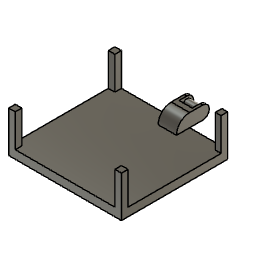
base-plate v2 (Autodesk Fusion 360 design; units mm, degrees)
Autodesk Fusion 360 part; units mm, degrees
sketch "Sketch1" plane through (0, 0, 0) normal (0, 0, 1) x (1, 0, 0)
  line L0 (0, 0) -> (76, 0)
  line L1 (76, 0) -> (76, 76)
  line L2 (76, 76) -> (0, 76)
  line L3 (0, 76) -> (0, 0)
  dimension "d1" = 76
  dimension "d2" = 76
  constraint horizontal L0
  constraint vertical L1
  constraint horizontal L2
  constraint vertical L3
  constraint coincident L0.start L3.end
  measures "d1" distance of L0.start L0.end
  measures "d2" distance of L0.start L2.end
extrude "Extrude1" add sketch "Sketch1" along normal blind 6.35
sketch "Sketch2" plane through (0, 0, 6.35) normal (0, 0, 1) x (-1, 0, 0)
  line L0 (0, -76) -> (0, 0)
  line L1 (0, 0) -> (-76, 0)
  line L2 (-76, 0) -> (-76, -76)
  line L3 (-76, -76) -> (0, -76)
  line L4 (-52, -66) -> (-38, -66)
  line L5 (-38, -66) -> (-38, -91)
  line L6 (-38, -91) -> (-52, -91)
  line L7 (-52, -91) -> (-52, -66)
  dimension "d5" = 14
  dimension "d6" = 25
  dimension "d7" = 24
  dimension "d8" = 10
  constraint horizontal L4
  constraint vertical L5
  constraint horizontal L6
  constraint vertical L7
  measures "d5" distance of L4.start L4.end
  measures "d6" distance of L4.start L6.end
  measures "d7" distance of L2 L7
  measures "d8" distance of L3 L4
extrude "Extrude2" add sketch "Sketch2" along normal blind 10 contours L3 L5 L6 L7 | L3 L4 L5 L7
fillet "Fillet1" radius 10 1 edges at (45, 66, 16.35)
fillet "Fillet2" radius 5 2 edges at (45, 91, 16.35) (45, 91, 6.35)
sketch "Sketch3" plane through (0, 0, 16.35) normal (0, 0, 1) x (-1, 0, 0)
  line L0 (-52, -86) -> (-38, -86)
  line L1 (-38, -86) -> (-38, -76)
  line L2 (-38, -76) -> (-52, -76)
  line L3 (-52, -76) -> (-52, -86)
  line L4 (-50, -80) -> (-40, -80)
  line L5 (-40, -80) -> (-40, -95)
  line L6 (-40, -95) -> (-50, -95)
  line L7 (-50, -95) -> (-50, -80)
  constraint horizontal L4
  constraint vertical L5
  constraint horizontal L6
  constraint vertical L7
extrude "Extrude3" cut sketch "Sketch3" against normal blind 20 contours L0 L4 L5 L7 | L0 L5 L6 L7
sketch "Sketch4" plane through (40, 0, 0) normal (1, 0, 0) x (0, 1, 0)
  line L0 (80, 6.35) -> (86, 6.35)
  arc A0 (86, 6.35) -> (86, 16.35) centre (86, 11.35) ccw
  line L1 (86, 16.35) -> (80, 16.35)
  line L2 (80, 16.35) -> (80, 6.35)
  circle A1 centre (86, 11.35) radius 3.25
  dimension "d17" = 6.5
  constraint concentric A0 A1
  measures "d17" diameter of A1
extrude "Extrude4" add sketch "Sketch4" along normal blind 10 contours A1
extrude "Extrude5" add 1 faces at (76, 25.3333, 2.1167) along direction (1, 0, 0) blind 5
extrude "Extrude6" add 1 faces at (0, 50.6667, 2.1167) along direction (-1, 0, 0) blind 5
extrude "Extrude7" add 1 faces at (23.6667, 0, 2.1167) along direction (0, -1, 0) blind 5
sketch "Sketch5" plane through (0, 0, 6.35) normal (0, 0, 1) x (-1, 0, 0)
  line L0 (-38, -66) -> (-38, -76)
  line L1 (-38, -76) -> (5, -76)
  line L2 (5, -76) -> (5, 5)
  line L3 (5, 5) -> (-81, 5)
  line L4 (-81, 5) -> (-81, -76)
  line L5 (-81, -76) -> (-52, -76)
  line L6 (-52, -76) -> (-52, -66)
  line L7 (-52, -66) -> (-38, -66)
  line L8 (-81, -76) -> (-76.6575, -76)
  line L9 (-76.6575, -76) -> (-76.6575, -71)
  line L10 (-76.6575, -71) -> (-81, -71)
  line L11 (-81, -71) -> (-81, -76)
  line L12 (5, -76) -> (0, -76)
  line L13 (0, -76) -> (0, -71)
  line L14 (0, -71) -> (5, -71)
  line L15 (5, -71) -> (5, -76)
  line L16 (5, 5) -> (0, 5)
  line L17 (0, 5) -> (0, 0)
  line L18 (0, 0) -> (5, 0)
  line L19 (5, 0) -> (5, 5)
  line L20 (-81, 5) -> (-76, 5)
  line L21 (-76, 5) -> (-76, 0)
  line L22 (-76, 0) -> (-81, 0)
  line L23 (-81, 0) -> (-81, 5)
  dimension "d26" = 5
  dimension "d27" = 5
  dimension "d28" = 5
  dimension "d29" = 5
  dimension "d30" = 5
  dimension "d31" = 5
  dimension "d32" = 5
  constraint horizontal L8
  constraint vertical L9
  constraint horizontal L10
  constraint vertical L11
  constraint coincident L4.end L5.start
  constraint horizontal L12
  constraint vertical L13
  constraint horizontal L14
  constraint vertical L15
  constraint coincident L1.end L2.start
  constraint horizontal L16
  constraint vertical L17
  constraint horizontal L18
  constraint vertical L19
  constraint coincident L2.end L3.start
  constraint horizontal L20
  constraint vertical L21
  constraint horizontal L22
  constraint vertical L23
  constraint coincident L3.end L4.start
  measures "d26" distance of L4.end L10.end
  measures "d27" distance of L1.end L12.end
  measures "d28" distance of L1.end L14.end
  measures "d29" distance of L2.end L16.end
  measures "d30" distance of L2.end L18.end
  measures "d31" distance of L3.end L20.end
  measures "d32" distance of L3.end L22.end
extrude "Extrude8" add sketch "Sketch5" along normal blind 25 contours L1 L2 L12 L13 L14 L15 | L4 L5 L8 L9 L10 L11 | L2 L3 L16 L17 L18 L19 | L3 L4 L20 L21 L22 L23
